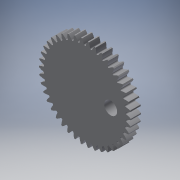
# Autodesk Inventor part: ServoGear
Saved by Autodesk Inventor 2019 (Build 230136000, 136)
## iProperties
Created: 2019-05-18
Part Number: ServoGear
Material: Generic
Document SubType Name: Modeling
Designer: Henry
Density: 1 g/cm^3
Appearance: Default
Author: Henry
Autodesk Inventor part; units mm, degrees
ref_plane "YZ Plane" through (0, 0, 0) normal (1, 0, 0) x (0, 1, 0)
ref_plane "XZ Plane" through (0, 0, 0) normal (0, 1, 0) x (-1, 0, 0)
ref_plane "XY Plane" through (0, 0, 0) normal (0, 0, 1) x (1, 0, 0)
sketch "Sketch1" plane through (0, 0, 0) normal (0, 0, 1) x (1, 0, 0)
  spline S0 degree 3 poles (-0.5507, 8.8829) (-0.5262, 8.8414) (-0.4774, 8.7585) (-0.41, 8.6306) (-0.358, 8.522) (-0.3195, 8.4337) (-0.2922, 8.3668) (-0.2666, 8.2992) (-0.243, 8.231) (-0.2212, 8.1621) (-0.206, 8.1038) (-0.1935, 8.0573) (-0.182, 8.0294) (-0.1701, 8.0084) (-0.1598, 7.9936) (-0.1484, 7.9795) (-0.1352, 7.9672) (-0.121, 7.9559) (-0.1054, 7.9467) (-0.0892, 7.9388) (-0.0718, 7.9337) (-0.0542, 7.9295) (-0.0301, 7.9282) (0, 7.929) (0.0301, 7.9282) (0.0542, 7.9295) (0.0718, 7.9337) (0.0892, 7.9388) (0.1054, 7.9467) (0.121, 7.9559) (0.1352, 7.9672) (0.1484, 7.9795) (0.1598, 7.9936) (0.1701, 8.0084) (0.182, 8.0294) (0.1935, 8.0573) (0.206, 8.1038) (0.2212, 8.1621) (0.243, 8.231) (0.2666, 8.2992) (0.2922, 8.3668) (0.3195, 8.4337) (0.358, 8.522) (0.41, 8.6306) (0.4774, 8.7585) (0.5262, 8.8414) (0.5507, 8.8829) knots 0 0 0 0 0.062504 0.125007 0.18751 0.218763 0.250016 0.281268 0.312521 0.343773 0.375025 0.390648 0.406265 0.414078 0.421886 0.429697 0.43751 0.44532 0.453133 0.460942 0.468752 0.476562 0.484373 0.5 0.515627 0.523438 0.531248 0.539058 0.546867 0.55468 0.56249 0.570303 0.578114 0.585922 0.593735 0.609352 0.624975 0.656227 0.687479 0.718732 0.749984 0.781237 0.81249 0.874993 0.937496 1 1 1 1
  circle A0 centre (0, 0) radius 7.9287 construction
  circle A1 centre (0, 0) radius 7.8934 construction
  circle A2 centre (0, 0) radius 8.4 construction
  circle A3 centre (0, 0) radius 8.9
  point P0 (-0.4784, 8.7579)
  point P1 (-0.4109, 8.6302)
  point P2 (-0.3487, 8.4998)
  point P3 (-0.3198, 8.4336)
  point P4 (-0.2925, 8.3667)
  point P5 (-0.267, 8.2991)
  point P6 (-0.2433, 8.2309)
  point P7 (-0.2218, 8.1619)
  point P8 (-0.2029, 8.0922)
  point P9 (-0.1928, 8.0575)
  point P10 (-0.1788, 8.0242)
  point P11 (-0.1699, 8.0086)
  point P12 (-0.1596, 7.9937)
  point P13 (-0.1481, 7.9798)
  point P14 (-0.135, 7.9674)
  point P15 (-0.1208, 7.9562)
  point P16 (-0.1053, 7.9469)
  point P17 (-0.089, 7.9393)
  point P18 (-0.0718, 7.9338)
  point P19 (-0.0541, 7.9301)
  point P20 (-0.0361, 7.9287)
  point P21 (0, 7.9287)
  point P22 (0.0361, 7.9287)
  point P23 (0.0541, 7.9301)
  point P24 (0.0718, 7.9338)
  point P25 (0.089, 7.9393)
  point P26 (0.1053, 7.9469)
  point P27 (0.1208, 7.9562)
  point P28 (0.135, 7.9674)
  point P29 (0.1481, 7.9798)
  point P30 (0.1596, 7.9937)
  point P31 (0.1699, 8.0086)
  point P32 (0.1788, 8.0242)
  point P33 (0.1928, 8.0575)
  point P34 (0.2029, 8.0922)
  point P35 (0.2218, 8.1619)
  point P36 (0.2433, 8.2309)
  point P37 (0.267, 8.2991)
  point P38 (0.2925, 8.3667)
  point P39 (0.3198, 8.4336)
  point P40 (0.3487, 8.4998)
  point P41 (0.4109, 8.6302)
  point P42 (0.4784, 8.7579)
  constraints: 4 centre point, 2 point on circle, 95 other
extrude "Extrusion1" add sketch "Sketch1" against normal blind 2
extrude "Extrusion2" cut sketch "Sketch1" against normal blind 2 contours A3 S0 picked at (-0.0366, 8.4917)
pattern_circular "Circular Pattern1" count 42 over 360 about axis through (0, 0, 0) along (0, 0, -1) of "Extrusion2"
sketch "Sketch3" plane through (0, 0, 0) normal (0, 0, 1) x (1, 0, 0)
  line L0 (0, 0) -> (5, 0)
  circle A0 centre (5, 0) radius 1.25
  dimension "d10" = 5
  dimension "d11" = 2.5
  constraints: 2 end point, 1 centre point, 1 coincident, 1 horizontal
  measures "d10" distance of L0.start L0.end
  measures "d11" diameter of A0
extrude "Extrusion4" cut sketch "Sketch3" against normal blind 2
equation "\"d0\" = FaceWidth"
equation "\"Module\" = 0.4"
equation "\"PressureAngle\" = 20deg"
equation "\"UnitProfileClearance\" = 0.25"
equation "\"UnitRoundRadius\" = 0.35"
equation "\"HeadDiameter\" = 17.8"
equation "\"RootDiameter\" = 15.8573"
equation "\"BaseDiameter\" = 15.78684"
equation "\"PitchDiameter\" = 16.8"
equation "\"FaceWidth\" = 2"
equation "\"HelixAngle\" = 0"
equation "\"UnitCorrection\" = 0.257289"
equation "\"UnitAddendumModification\" = 0.007289"
equation "\"CircularPitch\" = 1.25664"
equation "\"UnitBacklashShift\" = -0.185662"
equation "\"TotalToolShift\" = 0.02865"
equation "\"IsInternal\" = 0"
body "Solid1"
